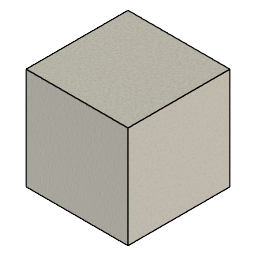
cube (Autodesk Fusion 360 design; units mm, degrees)
part number: 2025-09-13-11-51-53-799
Autodesk Fusion 360 part; units mm, degrees
sketch "草图3" plane through (0, 0, 0) normal (0, 0, 1) x (1, 0, 0)
  line L0 (20, 20) -> (-20, 20)
  line L1 (-20, 20) -> (-20, -20)
  line L2 (-20, -20) -> (20, -20)
  line L3 (20, -20) -> (20, 20)
  line L4 (20, 20) -> (-20, -20) construction
  line L5 (-20, 20) -> (20, -20) construction
  dimension "d2" = 40
  dimension "d3" = 40
  constraint horizontal L0
  constraint perpendicular L0 L1
  constraint parallel L0 L2
  constraint parallel L1 L3
  constraint coincident L4 origin
  constraint coincident L5 origin
  measures "d2" distance of L1.end L2.end
  measures "d3" distance of L0.end L1.end
extrude "拉伸1" add sketch "草图3" along normal blind 40
equation "d2 = side"
equation "d3 = side"
equation "side = 40 mm"
equation "d5 = side"
